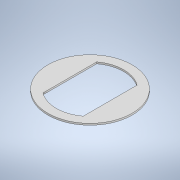
# Autodesk Inventor part: raceway_guard
Saved by Autodesk Inventor 2022 (Build 260153000, 153)
## iProperties
Created: 2022-03-15
Part Number: raceway_guard
Material: Generic
Document SubType Name: Modeling
Designer: kylem
Density: 1 g/cm^3
Appearance: Default
Author: kylem
Autodesk Inventor part; units mm, degrees
ref_plane "YZ Plane" through (0, 0, 0) normal (1, 0, 0) x (0, 1, 0)
ref_plane "XZ Plane" through (0, 0, 0) normal (0, 1, 0) x (-1, 0, 0)
ref_plane "XY Plane" through (0, 0, 0) normal (0, 0, 1) x (1, 0, 0)
sketch "Sketch1" plane through (0, 0, 0) normal (0, 1, 0) x (-1, 0, 0)
  circle A0 centre (0, 0) radius 25
  circle A1 centre (0, 0) radius 20
  line L0 (0, 0) -> (12, 0)
  line L1 (0, 0) -> (0, -2.5316)
  line L2 (12, 0) -> (12, -16)
  line L3 (12, -16) -> (12, 16)
  line L4 (-12, -16) -> (-12, 16)
  dimension "d0" = 50
  dimension "d1" = 40
  dimension "d3" = 12
  constraints: 10 end point, 2 centre point, 2 coincident, 2 point on circle, 2 symmetric about line, 2 vertical, 1 horizontal, 1 point on line
  measures "d0" diameter of A0
  measures "d1" diameter of A1
  measures "d3" distance of L0.start L0.end
extrude "Extrusion1" add sketch "Sketch1" along normal blind 1 contours A0 | A1 L2 L3 | L4 A1
body "Solid1"
